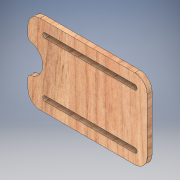
# Autodesk Inventor part: SuctionGrabberB
Saved by Autodesk Inventor 2019 (Build 230136000, 136)
## iProperties
Created: 2019-01-19
Part Number: SuctionGrabberB
Material: Wood (Birch)
Document SubType Name: Modeling
Designer: nxgam
Density: 0.55 g/cm^3
Appearance: Birch - Natural Polished
Author: nxgam
Autodesk Inventor part; units mm, degrees
ref_plane "YZ Plane" through (0, 0, 0) normal (1, 0, 0) x (0, 1, 0)
ref_plane "XZ Plane" through (0, 0, 0) normal (0, 1, 0) x (-1, 0, 0)
ref_plane "XY Plane" through (0, 0, 0) normal (0, 0, 1) x (1, 0, 0)
sketch "Sketch1" plane through (0, 0, 0) normal (0, 0, 1) x (1, 0, 0)
  line L0 (0, 0) -> (162.56, 0)
  line L1 (162.56, 0) -> (162.56, 81.28)
  line L2 (162.56, 81.28) -> (0, 81.28)
  line L3 (0, 81.28) -> (0, 0)
  dimension "d0" = 162.56
  dimension "d1" = 81.28
  constraints: 8 end point, 2 parallel, 1 horizontal, 1 perpendicular
  measures "d0" distance of L2.end L1.end
  measures "d1" distance of L1.end L0.end
extrude "Extrusion1" add sketch "Sketch1" along normal blind 5.08
sketch "Sketch2" plane through (0, 0, 5.08) normal (0, 0, 1) x (1, 0, 0)
  line L0 (0, 0) -> (162.56, 0) projected
  line L1 (162.56, 0) -> (162.56, 81.28) projected
  line L2 (162.56, 81.28) -> (0, 81.28) projected
  line L3 (0, 81.28) -> (0, 0) construction
  line L4 (0, 40.64) -> (162.56, 40.64) construction
  arc A0 (40.64, 55.88) -> (40.64, 25.4) centre (40.64, 40.64) ccw construction
  arc A1 (78.3143, 55.88) -> (40.64, 81.28) centre (40.64, 40.64) ccw construction
  line L5 (0, 81.28) -> (0, 0) projected
  line L6 (0, 0) -> (162.56, 0) projected
  line L7 (0, 81.28) -> (40.64, 81.28) construction
  line L8 (162.56, 81.28) -> (162.56, 0)
  line L9 (162.56, 0) -> (40.64, 0)
  line L10 (0, 0) -> (0, 40.64)
  line L11 (0, 40.64) -> (0, 81.28)
  line L12 (40.64, 0) -> (0, 0) construction
  line L13 (40.64, 81.28) -> (162.56, 81.28)
  line L14 (40.64, 25.4) -> (78.3143, 25.4)
  line L15 (40.64, 55.88) -> (78.3143, 55.88)
  line L16 (162.56, 0) -> (162.56, 81.28) projected
  line L17 (162.56, 23.2866) -> (162.56, 55.88)
  line L18 (40.64, 25.4) -> (78.3143, 25.4)
  line L19 (162.56, 25.4) -> (162.56, 55.88) construction
  line L20 (162.56, 55.88) -> (40.64, 55.88)
  line L21 (40.64, 55.88) -> (40.64, 40.64) construction
  arc A2 (55.88, 40.64) -> (40.64, 55.88) centre (40.64, 40.64) ccw
  arc A3 (40.64, 25.4) -> (55.88, 40.64) centre (40.64, 40.64) ccw
  arc A4 (81.28, 40.64) -> (78.3143, 55.88) centre (40.64, 40.64) ccw construction
  arc A5 (78.3143, 25.4) -> (81.28, 40.64) centre (40.64, 40.64) ccw construction
  arc A6 (40.64, 81.28) -> (2.9657, 55.88) centre (40.64, 40.64) ccw construction
  arc A7 (40.64, 0) -> (78.3143, 25.4) centre (40.64, 40.64) ccw construction
  arc A8 (0, 40.64) -> (2.9657, 25.4) centre (40.64, 40.64) ccw
  arc A9 (2.9657, 25.4) -> (40.64, 0) centre (40.64, 40.64) ccw
  arc A10 (2.9657, 55.88) -> (0, 40.64) centre (40.64, 40.64) ccw
  line L22 (78.3143, 55.88) -> (162.56, 55.88)
  line L23 (78.3143, 25.4) -> (162.56, 25.4)
  line L24 (78.3143, 25.4) -> (162.56, 25.4)
  line L25 (40.64, 81.28) -> (40.64, 55.88)
  line L26 (40.64, 40.64) -> (40.64, 25.4) construction
  line L27 (40.64, 55.88) -> (40.64, 40.64) construction
  line L28 (40.64, 25.4) -> (40.64, 0)
  line L29 (40.64, 40.64) -> (40.64, 25.4)
  dimension "d4" = 30.48
  constraints: 46 end point, 30 point on circle, 21 tangent, 11 centre point, 10 parallel, 7 point on line, 6 horizontal, 6 perpendicular, 4 vertical, 3 midpoint, 1 coincident, 1 collinear
  measures "d4" diameter of A0
extrude "Extrusion2" cut sketch "Sketch2" against normal blind 5.08 contours L28 L14 L23 L1 L0 | A3 A2 L15 L20 L1 L23 L14 | L2 L1 L20 L15 L25 keep common part
sketch "Sketch3" plane through (0, 0, 5.08) normal (0, 0, 1) x (1, 0, 0)
  line L0 (162.56, 0) -> (162.56, 81.28) projected
  line L1 (40.64, 0) -> (162.56, 0) projected
  line L2 (40.64, 40.64) -> (162.56, 40.64) construction
  line L3 (162.56, 40.64) -> (162.56, 25.4) construction
  line L4 (58.42, 68.58) -> (149.86, 68.58) construction
  line L5 (58.42, 66.08) -> (149.86, 66.08)
  line L6 (149.86, 71.08) -> (58.42, 71.08)
  arc A0 (58.42, 71.08) -> (58.42, 66.08) centre (58.42, 68.58) ccw
  arc A1 (149.86, 66.08) -> (149.86, 71.08) centre (149.86, 68.58) ccw
  line L7 (40.64, 55.88) -> (40.64, 81.28) construction
  line L8 (58.42, 12.7) -> (149.86, 12.7) construction
  line L9 (58.42, 15.2) -> (149.86, 15.2)
  line L10 (149.86, 10.2) -> (58.42, 10.2)
  arc A2 (58.42, 15.2) -> (58.42, 10.2) centre (58.42, 12.7) ccw
  arc A3 (149.86, 10.2) -> (149.86, 15.2) centre (149.86, 12.7) ccw
  line L11 (40.64, 0) -> (40.64, 25.4) projected
  line L12 (40.64, 55.88) -> (40.64, 81.28) projected
  arc A4 (40.64, 25.4) -> (40.64, 55.88) centre (40.64, 40.64) ccw projected
  line L13 (162.56, 81.28) -> (40.64, 81.28) projected
  point P0 (0, 0)
  point P1 (104.14, 68.58)
  point P2 (104.14, 12.7)
  dimension "d7" = 2.5
  dimension "d8" = 121.92
  dimension "d12" = 91.44
  dimension "d13" = 12.7
  constraints: 22 end point, 8 point on circle, 7 symmetric about line, 4 centre point, 4 tangent, 2 horizontal, 1 midpoint, 1 parallel, 1 perpendicular, 1 vertical, 2 other
  measures "d7" radius of A1
  measures "d8" distance between parallel lines of L0 L7
  measures "d12" distance of L4.start L4.end
  measures "d13" distance from line of L0 L4.end
extrude "Extrusion3" cut sketch "Sketch3" against normal blind 5.08 contours A0 L6 A1 L5 | L9 A3 L10 A2
fillet "Fillet1" radius 12.7 2 edges at (162.56, 0, 2.54) (162.56, 81.28, 2.54)
fillet "Fillet2" radius 12.7 2 edges at (40.64, 81.28, 2.54) (40.64, 0, 2.54)
fillet "Fillet3" radius 3.175 2 edges at (40.64, 55.88, 2.54) (40.64, 25.4, 2.54)
equation "\"d0\" = 2 * d1"
equation "\"d13\" = d11"
equation "\"d11\" = 0.5 * d10"
equation "\"d10\" = 25.4"
body "Solid1"
